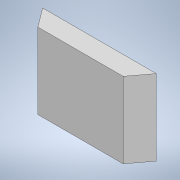
# Autodesk Inventor part: link_v2
Saved by Autodesk Inventor 2022 (Build 260153000, 153)
## iProperties
Created: 2022-05-21
Part Number: link_v2
Material: Generic
Document SubType Name: Modeling
Designer: kylem
Density: 1 g/cm^3
Appearance: Default
Author: kylem
Autodesk Inventor part; units mm, degrees
ref_plane "YZ Plane" through (0, 0, 0) normal (1, 0, 0) x (0, 1, 0)
ref_plane "XZ Plane" through (0, 0, 0) normal (0, 1, 0) x (-1, 0, 0)
ref_plane "XY Plane" through (0, 0, 0) normal (0, 0, 1) x (1, 0, 0)
sketch "Sketch1" plane through (0, 0, 0) normal (0, 1, 0) x (-1, 0, 0)
  line L0 (0, 0) -> (14, 0)
  line L1 (14, 0) -> (14, -2)
  line L2 (14, -2) -> (0, -2)
  line L3 (0, -2) -> (0, 0)
  line L4 (14, -1) -> (13, -1)
  line L5 (7, -2) -> (7, -1)
  circle A0 centre (13, -1) radius 0.5
  circle A1 centre (1, -1) radius 0.5
  dimension "d0" = 14
  dimension "d1" = 2
  dimension "d2" = 1
  dimension "d3" = 1
  constraints: 12 end point, 2 centre point, 2 horizontal, 2 midpoint, 2 parallel, 1 coincident, 1 perpendicular, 1 symmetric about line, 1 vertical, 1 other
  measures "d0" distance of L1.end L2.end
  measures "d1" distance of L0.end L1.end
  measures "d2" distance of L4.start L4.end
  measures "d3" diameter of A0
extrude "Extrusion1" add sketch "Sketch1" along normal blind 8
sketch "Sketch2" plane through (0, 8, 0) normal (0, 1, 0) x (1, 0, 0)
  circle A0 centre (-13, 1) radius 0.5 projected
  line L0 (-13, 1) -> (-11.5, 1)
  line L1 (-11.5, 1) -> (-11.5, 2)
  line L2 (0, 2) -> (-14, 2) projected
  line L3 (-11.5, 1) -> (-11.5, 0)
  line L4 (-14, 0) -> (0, 0) projected
  line L5 (-7, 2) -> (-7, 5.1392)
  line L6 (-13, 1) -> (-11.5, 2)
  line L7 (-13, 1) -> (-11.5, 0)
  circle A1 centre (-1, 1) radius 0.5
  line L8 (-1, 1) -> (-2.5, 1)
  line L9 (-2.5, 1) -> (-2.5, 2)
  line L10 (-14, 2) -> (0, 2)
  line L11 (-2.5, 1) -> (-2.5, 0)
  line L12 (0, 0) -> (-14, 0)
  line L13 (-1, 1) -> (-2.5, 2)
  line L14 (-1, 1) -> (-2.5, 0)
  line L15 (-11.5, 0) -> (-14, 0)
  line L16 (-14, 0) -> (-14, 2)
  line L17 (-14, 2) -> (-11.5, 2)
  line L18 (-11.5, 2) -> (-11.5, 0)
  line L19 (0, 0) -> (0, 2) projected
  line L20 (0, 0) -> (-2.5, 0)
  line L21 (-2.5, 0) -> (-2.5, 2)
  line L22 (-2.5, 2) -> (0, 2)
  line L23 (0, 2) -> (0, 0)
  point P0 (-12.584, 0.7226)
  point P1 (-12.584, 1.2774)
  point P2 (-1.416, 1.2774)
  point P3 (-1.416, 0.7226)
  dimension "d6" = 1.5
  constraints: 42 end point, 8 symmetric about line, 6 point on line, 4 parallel, 3 horizontal, 2 perpendicular, 2 vertical, 1 centre point, 1 midpoint, 1 other
  measures "d6" distance of L0.start L0.end
extrude "Extrusion2" add sketch "Sketch2" against normal blind 8 contours L0 L6 A0 | L0 L3 L7 A0 | A0 L7 L0 | A0 L6 L1 L0 | L11 L8 A1 L14 | L13 A1 L8 L9 | A1 L8 L14 | L13 L8 A1
extrude "Extrusion3" cut sketch "Sketch2" against normal blind 8 contours A0 L7 L4 L16 L2 L6 | L14 A1 L13 L2 L19 L4
sketch "Sketch3" plane through (0, 8, 0) normal (0, 1, 0) x (1, 0, 0)
  line L0 (-11.5, 2) -> (-13, 1) projected
  line L1 (-1, 1) -> (-2.5, 2) projected
  line L2 (-13, 1) -> (-1, 1)
  line L3 (-13, 1) -> (-11.5, 0) projected
  line L4 (-13, 1) -> (-0.4084, 1)
  line L5 (-0.4084, 1) -> (-0.4084, 3.5124)
  line L6 (-0.4084, 3.5124) -> (-13, 3.5124)
  line L7 (-13, 3.5124) -> (-13, 1)
  point P0 (0, 0)
  constraints: 10 end point, 2 horizontal, 2 parallel, 1 perpendicular
extrude "Extrusion4" cut sketch "Sketch3" against normal blind 8
sketch "Sketch4" plane through (0, 8, 0) normal (0, 1, 0) x (1, 0, 0)
  line L0 (-11.5, 0) -> (-11.5, -1)
  line L1 (-11.5, 0) -> (-13, 1) projected
  line L2 (-11.5, -1) -> (-13, 1)
  line L3 (-11.5, 0) -> (-2.5, 0) projected
  line L4 (-13, 1) -> (-11.5, 0)
  line L5 (-1, 1) -> (-13, 1) projected
  line L6 (-7, 1) -> (-7, 2.0592)
  line L7 (-2.5, 0) -> (-2.5, -1)
  line L8 (-2.5, 0) -> (-1, 1)
  line L9 (-2.5, -1) -> (-1, 1)
  line L10 (-1, 1) -> (-2.5, 0)
  line L11 (-11.5, -1) -> (-2.5, -1)
  line L12 (-11.5, 0) -> (-2.5, 0)
  point P0 (0, 0)
  dimension "d13" = 1
  constraints: 20 end point, 2 vertical, 1 horizontal, 1 midpoint, 1 symmetric about line
  measures "d13" distance of L0.start L0.end
extrude "Extrusion5" add sketch "Sketch4" against normal blind 8 contours L3 L7 L11 L0 | L0 L2 L1 | L8 L9 L7
body "Solid1"
